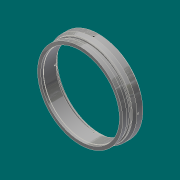
# Autodesk Inventor part: A1-19027-100-xx 32in Type B victaulic ring - thinned
Saved by Autodesk Inventor 2017.3 (Build 213256000, 256)
## iProperties
Created: 2013-12-16
Part Number: A1-19027-100-xx 32in Type B victaulic ring - thinned
Material: Steel, Mild
Document SubType Name: Modeling
Designer: Graeme_Van_Dongen
Density: 7.86 g/cm^3
Appearance: Steel
Description: 32" TYPE B VICTAULIC RING FOR STYLE 275 COUPLING, A105N, CUSTOM INVERTED B
Mass: 109782 g
Surface Area: 13413.1 cm^2
Volume: 13967.2 cm^3
Author: Graeme_Van_Dongen
Autodesk Inventor part; units mm, degrees
ref_plane "YZ Plane" through (0, 0, 0) normal (1, 0, 0) x (0, 1, 0)
ref_plane "XY Plane" through (0, 0, 0) normal (0, 0, 1) x (1, 0, 0)
sketch "Sketch1" plane through (0, 0, 0) normal (1, 0, 0) x (0, 1, 0)
  line L0 (401.32, 0) -> (401.32, 127)
  line L1 (404.8125, 152.4) -> (438.15, 152.4)
  line L2 (438.15, 152.4) -> (438.15, 109.622)
  line L3 (438.15, 109.622) -> (425.45, 107.95)
  line L4 (425.45, 107.95) -> (425.45, 73.66)
  line L5 (425.45, 73.66) -> (438.15, 70.9026)
  line L6 (438.15, 70.9026) -> (438.15, 60.96)
  line L7 (0, -91.44) -> (0, 193.04) projected
  arc A0 (438.15, 60.96) -> (439.8515, 54.61) centre (450.85, 60.96) ccw
  line L8 (439.8515, 54.61) -> (457.2, 24.5615)
  line L9 (457.2, 24.5615) -> (457.2, -36.2011)
  line L10 (457.2, -36.2011) -> (442.9125, -44.45)
  line L11 (442.9125, -44.45) -> (439.7375, -44.45)
  line L12 (439.7375, -44.45) -> (439.7375, -50.8)
  line L13 (439.7375, -50.8) -> (438.15, -50.8)
  line L14 (438.15, -50.8) -> (438.15, -43.4959)
  arc A1 (438.15, -43.4959) -> (436.4485, -37.1459) centre (425.45, -43.4959) ccw
  line L15 (407.67, 0) -> (401.32, 0)
  line L16 (401.32, 127) -> (404.8125, 127)
  line L17 (404.8125, 127) -> (404.8125, 152.4)
  line L18 (436.4485, -37.1459) -> (418.6685, -6.35)
  arc A2 (418.6685, -6.35) -> (407.67, 0) centre (407.67, -12.7) ccw
  point P0 (0, 0)
  point P1 (415.0023, 0)
  dimension "d0" = 401.32
  dimension "d13" = 425.45
  dimension "d14" = 438.15
  dimension "d16" = 44.45
  dimension "d17" = 34.29
  dimension "d18" = 7.5
  dimension "d19" = 12.25
  dimension "d32" = 457.2
  dimension "d33" = 14.2875
  dimension "d34" = 3.175
  dimension "d35" = 1.5875
  dimension "d36" = 12.7
  dimension "d37" = 30
  dimension "d38" = 203.2
  dimension "d39" = 6.35
  dimension "d40" = 12.7
  dimension "d41" = 60
  dimension "d42" = 12.7
  dimension "d72" = 152.4
  dimension "d75" = 25.4
  dimension "d78" = 30
  dimension "d80" = 0.9541
  dimension "d81" = 12.7
  dimension "d82" = 6.35
  dimension "d84" = 404.8125
  constraints: 36 end point, 7 perpendicular, 6 point on circle, 6 tangent, 3 centre point, 3 parallel, 3 point on line, 2 vertical, 1 collinear, 1 horizontal
  measures "d0" distance from line of point (0, 0) L0
  measures "d13" distance from line of point (0, 0) L4
  measures "d14" distance from line of point (0, 0) L6
  measures "d16" distance from line of L3.end L1
  measures "d17" distance of L3.end L4.end
  measures "d18" angle of L1 L3
  measures "d19" angle of L5 L1
  measures "d32" distance between parallel lines of L7 L9
  measures "d33" horizontal distance of L9.end L10.end
  measures "d34" distance of L10.end L11.end
  measures "d35" distance of L12.end L13.end
  measures "d36" radius of A1
  measures "d37" angle of L11 L10
  measures "d38" distance between parallel lines of L13 L1
  measures "d39" distance of L11.end L12.end
  measures "d40" radius of A0
  measures "d41" angle of L1 L8
  measures "d42" vertical distance of L4.end A0.centre
  measures "d72" distance between parallel lines of L15 L1
  measures "d75" distance of L16.end L1.start
  measures "d78" angle of L14 L18
  measures "d80" distance from line of A1.centre L11
  measures "d81" radius of A2
  measures "d82" distance of L15.start L0.start
  measures "d84" distance between parallel lines of L7 L17
revolve "Revolution1" add sketch "Sketch1" angle 360 about axis through (0, 0, -10) along (0, 0, 1)
chamfer "Chamfer2" distance 0.7937 angle 45 1 edges at (0, -401.32, 127)
fillet "Fillet1" radius 0.7937 1 edges at (0, -404.8125, 127)
ref_plane "Work Plane1" through (0, 457.2, -5.8198) normal (0, 1, 0) x (-1, 0, 0)
sketch "Sketch5" plane through (0, 457.2, -5.8198) normal (0, 1, 0) x (-1, 0, 0)
  line L0 (-438.15, 158.2198) -> (438.15, 158.2198) construction
  point P0 (0, 5.8198)
  point P1 (0, 18.5198)
  point P2 (-415.1313, -15.914)
  point P3 (415.1313, -15.914)
  dimension "d83" = 139.7
  constraints: 1 vertical alignment
  measures "d83" distance from line of point (0, 18.52) L0
hole "Hole1" at (0, 457.2, 12.7) direction (0, -1, 0) diameter 17.4752 depth 22.6314 tip angle 118 taper from width 18.3226 to width 17.4752 over 13.5636 thread size "1/2" designation "1/2 - 14 NPT" standard "NPT"
hole "Hole2" at (0, 457.2, 12.7) direction (0, -1, 0) diameter 10.5918 depth 76.2 tip angle 118 thread size "1/2-13 UNC" class "2B" standard "ANSI Unified Screw Threads"
pattern_circular "Circular Pattern2" count 4 over 360 about axis through (0, 0, -5.8198) along (0, 0, -1) of "Hole1", "Hole2"
body "Solid1"
